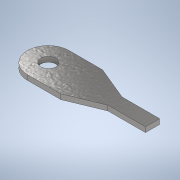
# Autodesk Inventor part: Negative Pin
Saved by Autodesk Inventor 2020 (Build 240168000, 168)
## iProperties
Created: 2021-12-31
Part Number: Negative Pin
Material: Copper, Alloy
Document SubType Name: Modeling
Designer: robur
Density: 8.92 g/cm^3
Appearance: Steel Galvanized
Author: robur
Autodesk Inventor part; units mm, degrees
ref_plane "YZ Plane" through (0, 0, 0) normal (1, 0, 0) x (0, 1, 0)
ref_plane "XZ Plane" through (0, 0, 0) normal (0, 1, 0) x (-1, 0, 0)
ref_plane "XY Plane" through (0, 0, 0) normal (0, 0, 1) x (1, 0, 0)
sketch "Sketch2" plane through (0, 0, 0) normal (0, 1, 0) x (-1, 0, 0)
  line L0 (-7.5, 0.85) -> (-7.5, -0.85)
  line L1 (1, -2.5) -> (5, -2.5)
  line L2 (7.5, 2.5) -> (-7.5, -2.5) construction
  line L3 (-7.5, 2.5) -> (7.5, -2.5) construction
  arc A0 (5, -2.5) -> (5, 2.5) centre (5, 0) ccw
  circle A1 centre (5, 0) radius 0.9
  line L4 (-3, 0.85) -> (-7.5, 0.85)
  line L5 (-7.5, 0.85) -> (-7.5, -0.85)
  line L6 (-7.5, -0.85) -> (-3, -0.85)
  line L7 (1, 2.5) -> (-3, 0.85)
  line L8 (-3, -0.85) -> (1, -2.5)
  line L9 (5, 2.5) -> (1, 2.5)
  point P0 (0, 0)
  dimension "d3" = 1.8
  constraints: 20 end point, 2 centre point, 2 horizontal, 2 midpoint, 2 parallel, 2 perpendicular, 2 point on circle
  measures "d3" diameter of A1
extrude "Extrusion1" add sketch "Sketch2" along normal blind 0.6
sketch "Sketch3" plane through (0, 0, 0) normal (0, -1, 0) x (1, 0, 0)
  line L0 (-2.413, -1.1278) -> (-2.413, 1.9227) construction
  line L1 (-2.413, 1.9227) -> (-0.0196, 1.9227) construction
  line L2 (-0.0196, 1.9227) -> (-0.0196, -1.1278) construction
  line L3 (-0.0196, -1.1278) -> (-2.413, -1.1278) construction
  line L4 (-2.1487, 1.1916) -> (-2.1487, -1.1599)
  line L5 (-2.1487, -1.1599) -> (-2.413, -1.1599)
  line L6 (-2.413, -1.1599) -> (-2.413, 1.1916)
  line L7 (-2.413, 1.1916) -> (-2.1487, 1.1916)
  point P0 (0, 0)
  constraints: 2 other
extrude "Extrusion2" add sketch "Sketch3" along normal blind 0.1
body "Solid1"
